Autodesk Fusion 360 part; units mm, degrees
note: some values were not read from the file. Set by a fixed rule: which sketch regions a step uses.
(part 2 of 3)
  arc A535 (3.7573, 18.103) -> (3.7523, 18.103) centre (3.7548, 18.103) ccw
  line L150 (3.7548, 18.103) -> (3.9714, 17.985)
  arc A536 (0.2852, 36.0425) -> (0.2802, 36.0425) centre (0.2827, 36.0425) ccw
  arc A537 (3.5261, 18.189) -> (3.5211, 18.189) centre (3.5236, 18.189) ccw
  arc A538 (3.048, 18.259) -> (3.043, 18.259) centre (3.0455, 18.259) ccw
  line L151 (1.2615, 18.409) -> (1.5123, 18.324)
  line L152 (1.5123, 18.324) -> (1.7721, 18.272)
  arc A539 (0.163, 35.8049) -> (0.168, 35.8049) centre (0.1655, 35.8049) ccw
  arc A540 (2.0389, 18.255) -> (2.0339, 18.255) centre (2.0364, 18.255) ccw
  arc A541 (1.0214, 18.526) -> (1.0264, 18.526) centre (1.0239, 18.526) ccw
  arc A542 (1.7696, 18.272) -> (1.7746, 18.272) centre (1.7721, 18.272) ccw
  arc A543 (0.0779, 35.5541) -> (0.0829, 35.5541) centre (0.0804, 35.5541) ccw
  arc A544 (0.0139, 20.28) -> (0.0089, 20.28) centre (0.0114, 20.28) ccw
  arc A545 (3.5261, 18.189) -> (3.5211, 18.189) centre (3.5236, 18.189) ccw
  arc A546 (3.0389, 18.255) -> (3.0339, 18.255) centre (3.0364, 18.255) ccw
  arc A547 (3.7573, 18.103) -> (3.7523, 18.103) centre (3.7548, 18.103) ccw
  arc A548 (3.043, 18.259) -> (3.048, 18.259) centre (3.0455, 18.259) ccw
  arc A549 (3.0339, 18.255) -> (3.0389, 18.255) centre (3.0364, 18.255) ccw
  arc A550 (1.0264, 18.526) -> (1.0214, 18.526) centre (1.0239, 18.526) ccw
  arc A551 (1.264, 18.409) -> (1.259, 18.409) centre (1.2615, 18.409) ccw
  arc A552 (2.0389, 18.255) -> (2.0339, 18.255) centre (2.0364, 18.255) ccw
  arc A553 (3.9739, 17.985) -> (3.9689, 17.985) centre (3.9714, 17.985) ccw
  arc A554 (3.9689, 17.985) -> (3.9739, 17.985) centre (3.9714, 17.985) ccw
  arc A555 (3.285, 18.242) -> (3.28, 18.242) centre (3.2825, 18.242) ccw
  arc A556 (4.1664, 17.837) -> (4.1714, 17.837) centre (4.1689, 17.837) ccw
  arc A557 (4.1714, 17.837) -> (4.1664, 17.837) centre (4.1689, 17.837) ccw
  arc A558 (0.8012, 18.6735) -> (0.8062, 18.6735) centre (0.8037, 18.6735) ccw
  arc A559 (0.8062, 18.6735) -> (0.8012, 18.6735) centre (0.8037, 18.6735) ccw
  line L153 (3.9714, 17.985) -> (4.1689, 17.837)
  arc A560 (1.259, 18.409) -> (1.264, 18.409) centre (1.2615, 18.409) ccw
  arc A561 (3.9739, 17.985) -> (3.9689, 17.985) centre (3.9714, 17.985) ccw
  arc A562 (4.1714, 17.837) -> (4.1664, 17.837) centre (4.1689, 17.837) ccw
  arc A563 (4.607, 17.248) -> (4.612, 17.248) centre (4.6095, 17.248) ccw
  line L154 (4.6958, 16.043) -> (4.7482, 16.284)
  arc A564 (1.0264, 18.526) -> (1.0214, 18.526) centre (1.0239, 18.526) ccw
  arc A565 (4.3459, 15.397) -> (4.3409, 15.397) centre (4.3434, 15.397) ccw
  arc A566 (4.6933, 17.017) -> (4.6983, 17.017) centre (4.6958, 17.017) ccw
  arc A567 (4.3409, 15.397) -> (4.3459, 15.397) centre (4.3434, 15.397) ccw
  line L155 (3.0455, 18.259) -> (3.2825, 18.242)
  arc A568 (1.5148, 18.324) -> (1.5098, 18.324) centre (1.5123, 18.324) ccw
  arc A569 (1.7696, 18.272) -> (1.7746, 18.272) centre (1.7721, 18.272) ccw
  arc A570 (1.5098, 18.324) -> (1.5148, 18.324) centre (1.5123, 18.324) ccw
  arc A571 (4.6983, 17.017) -> (4.6933, 17.017) centre (4.6958, 17.017) ccw
  arc A572 (4.607, 15.812) -> (4.612, 15.812) centre (4.6095, 15.812) ccw
  arc A573 (4.6983, 16.043) -> (4.6933, 16.043) centre (4.6958, 16.043) ccw
  arc A574 (4.1664, 15.223) -> (4.1714, 15.223) centre (4.1689, 15.223) ccw
  arc A575 (4.7633, 16.53) -> (4.7683, 16.53) centre (4.7658, 16.53) ccw
  arc A576 (3.28, 18.242) -> (3.285, 18.242) centre (3.2825, 18.242) ccw
  line L156 (4.7482, 16.776) -> (4.7658, 16.53)
  arc A577 (4.607, 15.812) -> (4.612, 15.812) centre (4.6095, 15.812) ccw
  arc A578 (0.602, 18.8481) -> (0.607, 18.8481) centre (0.6045, 18.8481) ccw
  arc A579 (4.7683, 16.53) -> (4.7633, 16.53) centre (4.7658, 16.53) ccw
  arc A580 (4.7507, 16.776) -> (4.7457, 16.776) centre (4.7482, 16.776) ccw
  arc A581 (4.4938, 15.595) -> (4.4888, 15.595) centre (4.4913, 15.595) ccw
  arc A582 (4.3409, 17.663) -> (4.3459, 17.663) centre (4.3434, 17.663) ccw
  arc A583 (3.9739, 15.075) -> (3.9689, 15.075) centre (3.9714, 15.075) ccw
  line L157 (4.4913, 15.595) -> (4.6095, 15.812)
  arc A584 (4.1664, 15.223) -> (4.1714, 15.223) centre (4.1689, 15.223) ccw
  arc A585 (4.6933, 16.043) -> (4.6983, 16.043) centre (4.6958, 16.043) ccw
  arc A586 (4.4888, 15.595) -> (4.4938, 15.595) centre (4.4913, 15.595) ccw
  arc A587 (4.7683, 16.53) -> (4.7633, 16.53) centre (4.7658, 16.53) ccw
  arc A588 (4.3409, 15.397) -> (4.3459, 15.397) centre (4.3434, 15.397) ccw
  line L158 (4.4913, 17.465) -> (4.6095, 17.248)
  arc A589 (2.0339, 18.255) -> (2.0389, 18.255) centre (2.0364, 18.255) ccw
  line L159 (3.2825, 18.242) -> (3.5236, 18.189)
  arc A590 (4.7457, 16.776) -> (4.7507, 16.776) centre (4.7482, 16.776) ccw
  arc A591 (4.4888, 15.595) -> (4.4938, 15.595) centre (4.4913, 15.595) ccw
  line L160 (4.6095, 17.248) -> (4.6958, 17.017)
  arc A592 (4.7633, 16.53) -> (4.7683, 16.53) centre (4.7658, 16.53) ccw
  arc A593 (4.612, 17.248) -> (4.607, 17.248) centre (4.6095, 17.248) ccw
  arc A594 (4.7507, 16.284) -> (4.7457, 16.284) centre (4.7482, 16.284) ccw
  arc A595 (4.4938, 17.465) -> (4.4888, 17.465) centre (4.4913, 17.465) ccw
  line L161 (4.3434, 17.663) -> (4.4913, 17.465)
  arc A596 (4.6983, 17.017) -> (4.6933, 17.017) centre (4.6958, 17.017) ccw
  arc A597 (4.6933, 17.017) -> (4.6983, 17.017) centre (4.6958, 17.017) ccw
  line L162 (4.1689, 17.837) -> (4.3434, 17.663)
  arc A598 (4.7507, 16.284) -> (4.7457, 16.284) centre (4.7482, 16.284) ccw
  arc A599 (4.4938, 15.595) -> (4.4888, 15.595) centre (4.4913, 15.595) ccw
  arc A600 (4.3459, 15.397) -> (4.3409, 15.397) centre (4.3434, 15.397) ccw
  arc A601 (4.1714, 15.223) -> (4.1664, 15.223) centre (4.1689, 15.223) ccw
  arc A602 (4.612, 15.812) -> (4.607, 15.812) centre (4.6095, 15.812) ccw
  arc A603 (4.612, 15.812) -> (4.607, 15.812) centre (4.6095, 15.812) ccw
  line L163 (3.9714, 15.075) -> (4.1689, 15.223)
  arc A604 (3.9689, 15.075) -> (3.9739, 15.075) centre (3.9714, 15.075) ccw
  arc A605 (4.4888, 17.465) -> (4.4938, 17.465) centre (4.4913, 17.465) ccw
  arc A606 (3.28, 18.242) -> (3.285, 18.242) centre (3.2825, 18.242) ccw
  line L164 (4.3434, 15.397) -> (4.4913, 15.595)
  arc A607 (4.3409, 17.663) -> (4.3459, 17.663) centre (4.3434, 17.663) ccw
  arc A608 (4.3459, 17.663) -> (4.3409, 17.663) centre (4.3434, 17.663) ccw
  arc A609 (4.7457, 16.284) -> (4.7507, 16.284) centre (4.7482, 16.284) ccw
  arc A610 (4.612, 17.248) -> (4.607, 17.248) centre (4.6095, 17.248) ccw
  arc A611 (4.4888, 17.465) -> (4.4938, 17.465) centre (4.4913, 17.465) ccw
  line L165 (4.6095, 15.812) -> (4.6958, 16.043)
  arc A612 (3.285, 18.242) -> (3.28, 18.242) centre (3.2825, 18.242) ccw
  line L166 (4.1689, 15.223) -> (4.3434, 15.397)
  arc A613 (4.4938, 17.465) -> (4.4888, 17.465) centre (4.4913, 17.465) ccw
  line L167 (4.7482, 16.284) -> (4.7658, 16.53)
  arc A614 (4.3459, 17.663) -> (4.3409, 17.663) centre (4.3434, 17.663) ccw
  arc A615 (4.7457, 16.284) -> (4.7507, 16.284) centre (4.7482, 16.284) ccw
  arc A616 (4.607, 17.248) -> (4.612, 17.248) centre (4.6095, 17.248) ccw
  arc A617 (4.6983, 16.043) -> (4.6933, 16.043) centre (4.6958, 16.043) ccw
  line L168 (4.6958, 17.017) -> (4.7482, 16.776)
  arc A618 (4.7507, 16.776) -> (4.7457, 16.776) centre (4.7482, 16.776) ccw
  arc A619 (4.7457, 16.776) -> (4.7507, 16.776) centre (4.7482, 16.776) ccw
  arc A620 (4.1664, 17.837) -> (4.1714, 17.837) centre (4.1689, 17.837) ccw
  arc A621 (4.6933, 16.043) -> (4.6983, 16.043) centre (4.6958, 16.043) ccw
  line L169 (1.2615, 14.651) -> (1.5123, 14.736)
  arc A622 (1.259, 14.651) -> (1.264, 14.651) centre (1.2615, 14.651) ccw
  arc A623 (1.5098, 14.736) -> (1.5148, 14.736) centre (1.5123, 14.736) ccw
  arc A624 (3.7573, 14.957) -> (3.7523, 14.957) centre (3.7548, 14.957) ccw
  arc A625 (1.7746, 14.788) -> (1.7696, 14.788) centre (1.7721, 14.788) ccw
  arc A626 (2.0389, 14.805) -> (2.0339, 14.805) centre (2.0364, 14.805) ccw
  arc A627 (1.5148, 14.736) -> (1.5098, 14.736) centre (1.5123, 14.736) ccw
  arc A628 (1.259, 14.651) -> (1.264, 14.651) centre (1.2615, 14.651) ccw
  arc A629 (0.8062, 14.387) -> (0.8012, 14.387) centre (0.8037, 14.387) ccw
  arc A630 (56.082, 29.6125) -> (56.077, 29.6125) centre (56.0795, 29.6125) ccw
  arc A631 (56.2584, 29.5441) -> (56.2534, 29.5441) centre (56.2559, 29.5441) ccw
  arc A632 (56.4393, 29.5094) -> (56.4443, 29.5094) centre (56.4418, 29.5094) ccw
  arc A633 (55.5089, 30.53) -> (55.5139, 30.53) centre (55.5114, 30.53) ccw
  arc A634 (56.4393, 29.5094) -> (56.4443, 29.5094) centre (56.4418, 29.5094) ccw
  arc A635 (55.5139, 32.53) -> (55.5089, 32.53) centre (55.5114, 32.53) ccw
  arc A636 (56.4443, 29.5094) -> (56.4393, 29.5094) centre (56.4418, 29.5094) ccw
  line L170 (55.5289, 32.7183) -> (55.5806, 32.9003)
  line L171 (55.5114, 32.53) -> (55.5289, 32.7183)
  arc A637 (55.6624, 33.0696) -> (55.6674, 33.0696) centre (55.6649, 33.0696) ccw
  arc A638 (55.5831, 32.9003) -> (55.5781, 32.9003) centre (55.5806, 32.9003) ccw
  arc A639 (55.5781, 30.1597) -> (55.5831, 30.1597) centre (55.5806, 30.1597) ccw
  arc A640 (55.7814, 29.8395) -> (55.7764, 29.8395) centre (55.7789, 29.8395) ccw
  arc A641 (55.7764, 29.8395) -> (55.7814, 29.8395) centre (55.7789, 29.8395) ccw
  arc A642 (55.5831, 30.1597) -> (55.5781, 30.1597) centre (55.5806, 30.1597) ccw
  arc A643 (55.6674, 29.9904) -> (55.6624, 29.9904) centre (55.6649, 29.9904) ccw
  arc A644 (55.5139, 30.53) -> (55.5089, 30.53) centre (55.5114, 30.53) ccw
  arc A645 (55.5139, 30.53) -> (55.5089, 30.53) centre (55.5114, 30.53) ccw
  arc A646 (55.5314, 32.7183) -> (55.5264, 32.7183) centre (55.5289, 32.7183) ccw
  arc A647 (55.5831, 30.1597) -> (55.5781, 30.1597) centre (55.5806, 30.1597) ccw
  arc A648 (55.6624, 29.9904) -> (55.6674, 29.9904) centre (55.6649, 29.9904) ccw
  arc A649 (55.6674, 29.9904) -> (55.6624, 29.9904) centre (55.6649, 29.9904) ccw
  line L172 (55.6649, 29.9904) -> (55.7789, 29.8395)
  line L173 (55.9187, 29.712) -> (56.0795, 29.6125)
  arc A650 (56.077, 29.6125) -> (56.082, 29.6125) centre (56.0795, 29.6125) ccw
  line L174 (56.4418, 29.5094) -> (56.631, 29.5094)
  arc A651 (55.5314, 30.3417) -> (55.5264, 30.3417) centre (55.5289, 30.3417) ccw
  arc A652 (55.6624, 29.9904) -> (55.6674, 29.9904) centre (55.6649, 29.9904) ccw
  arc A653 (55.5139, 32.53) -> (55.5089, 32.53) centre (55.5114, 32.53) ccw
  line L175 (55.5114, 30.53) -> (55.5114, 32.53)
  arc A654 (55.5089, 32.53) -> (55.5139, 32.53) centre (55.5114, 32.53) ccw
  arc A655 (55.5264, 32.7183) -> (55.5314, 32.7183) centre (55.5289, 32.7183) ccw
  arc A656 (55.7764, 29.8395) -> (55.7814, 29.8395) centre (55.7789, 29.8395) ccw
  arc A657 (55.5264, 30.3417) -> (55.5314, 30.3417) centre (55.5289, 30.3417) ccw
  arc A658 (55.5314, 32.7183) -> (55.5264, 32.7183) centre (55.5289, 32.7183) ccw
  line L176 (55.7789, 29.8395) -> (55.9187, 29.712)
  arc A659 (55.7814, 29.8395) -> (55.7764, 29.8395) centre (55.7789, 29.8395) ccw
  line L177 (55.5289, 30.3417) -> (55.5806, 30.1597)
  arc A660 (56.2534, 29.5441) -> (56.2584, 29.5441) centre (56.2559, 29.5441) ccw
  arc A661 (56.4443, 29.5094) -> (56.4393, 29.5094) centre (56.4418, 29.5094) ccw
  line L178 (55.5806, 30.1597) -> (55.6649, 29.9904)
  line L179 (55.5114, 30.53) -> (55.5289, 30.3417)
  arc A662 (55.5781, 30.1597) -> (55.5831, 30.1597) centre (55.5806, 30.1597) ccw
  arc A663 (55.9162, 29.712) -> (55.9212, 29.712) centre (55.9187, 29.712) ccw
  arc A664 (55.9212, 29.712) -> (55.9162, 29.712) centre (55.9187, 29.712) ccw
  arc A665 (56.6335, 29.5094) -> (56.6285, 29.5094) centre (56.631, 29.5094) ccw
  arc A666 (56.6285, 29.5094) -> (56.6335, 29.5094) centre (56.631, 29.5094) ccw
  line L180 (56.2559, 29.5441) -> (56.4418, 29.5094)
  arc A667 (56.082, 29.6125) -> (56.077, 29.6125) centre (56.0795, 29.6125) ccw
  arc A668 (55.9212, 29.712) -> (55.9162, 29.712) centre (55.9187, 29.712) ccw
  arc A669 (56.2534, 29.5441) -> (56.2584, 29.5441) centre (56.2559, 29.5441) ccw
  arc A670 (55.5314, 30.3417) -> (55.5264, 30.3417) centre (55.5289, 30.3417) ccw
  line L181 (55.5806, 32.9003) -> (55.6649, 33.0696)
  arc A671 (55.5264, 30.3417) -> (55.5314, 30.3417) centre (55.5289, 30.3417) ccw
  arc A672 (55.5089, 30.53) -> (55.5139, 30.53) centre (55.5114, 30.53) ccw
  arc A673 (56.2584, 29.5441) -> (56.2534, 29.5441) centre (56.2559, 29.5441) ccw
  arc A674 (56.6285, 29.5094) -> (56.6335, 29.5094) centre (56.631, 29.5094) ccw
  arc A675 (55.9162, 29.712) -> (55.9212, 29.712) centre (55.9187, 29.712) ccw
  arc A676 (56.077, 29.6125) -> (56.082, 29.6125) centre (56.0795, 29.6125) ccw
  line L182 (56.631, 29.5094) -> (56.8169, 29.5441)
  arc A677 (55.5089, 32.53) -> (55.5139, 32.53) centre (55.5114, 32.53) ccw
  line L183 (56.0795, 29.6125) -> (56.2559, 29.5441)
  arc A678 (57.2914, 29.8395) -> (57.2964, 29.8395) centre (57.2939, 29.8395) ccw
  arc A679 (57.2964, 29.8395) -> (57.2914, 29.8395) centre (57.2939, 29.8395) ccw
  arc A680 (57.4897, 30.1597) -> (57.4947, 30.1597) centre (57.4922, 30.1597) ccw
  arc A681 (57.1566, 29.712) -> (57.1516, 29.712) centre (57.1541, 29.712) ccw
  arc A682 (57.4104, 29.9904) -> (57.4054, 29.9904) centre (57.4079, 29.9904) ccw
  arc A683 (57.4947, 30.1597) -> (57.4897, 30.1597) centre (57.4922, 30.1597) ccw
  arc A684 (57.5464, 30.3417) -> (57.5414, 30.3417) centre (57.5439, 30.3417) ccw
  arc A685 (57.1516, 29.712) -> (57.1566, 29.712) centre (57.1541, 29.712) ccw
  arc A686 (107.0509, 0.276) -> (107.0459, 0.276) centre (107.0484, 0.276) ccw
  arc A687 (64.5089, 30.53) -> (64.5139, 30.53) centre (64.5114, 30.53) ccw
  arc A688 (57.1516, 29.712) -> (57.1566, 29.712) centre (57.1541, 29.712) ccw
  arc A689 (117.4659, 17.248) -> (117.4609, 17.248) centre (117.4634, 17.248) ccw
  line L184 (57.2939, 29.8395) -> (57.4079, 29.9904)
  arc A690 (117.5789, 17.465) -> (117.5839, 17.465) centre (117.5814, 17.465) ccw
  arc A691 (117.5839, 17.465) -> (117.5789, 17.465) centre (117.5814, 17.465) ccw
  arc A692 (56.9958, 29.6125) -> (56.9908, 29.6125) centre (56.9933, 29.6125) ccw
  line L185 (56.631, 33.5506) -> (56.8169, 33.5159)
  arc A693 (56.8144, 29.5441) -> (56.8194, 29.5441) centre (56.8169, 29.5441) ccw
  arc A694 (57.4104, 29.9904) -> (57.4054, 29.9904) centre (57.4079, 29.9904) ccw
  arc A695 (56.6285, 33.5506) -> (56.6335, 33.5506) centre (56.631, 33.5506) ccw
  arc A696 (56.6335, 33.5506) -> (56.6285, 33.5506) centre (56.631, 33.5506) ccw
  arc A697 (56.8144, 33.5159) -> (56.8194, 33.5159) centre (56.8169, 33.5159) ccw
  arc A698 (57.4054, 29.9904) -> (57.4104, 29.9904) centre (57.4079, 29.9904) ccw
  arc A699 (57.4897, 30.1597) -> (57.4947, 30.1597) centre (57.4922, 30.1597) ccw
  arc A700 (57.4947, 30.1597) -> (57.4897, 30.1597) centre (57.4922, 30.1597) ccw
  line L186 (57.5439, 30.3417) -> (57.5614, 30.53)
  arc A701 (57.2964, 29.8395) -> (57.2914, 29.8395) centre (57.2939, 29.8395) ccw
  line L187 (57.4922, 30.1597) -> (57.5439, 30.3417)
  line L188 (107.0484, 0.276) -> (107.2694, 0.423)
  arc A702 (57.5414, 30.3417) -> (57.5464, 30.3417) centre (57.5439, 30.3417) ccw
  line L189 (57.4079, 29.9904) -> (57.4922, 30.1597)
  arc A703 (56.9908, 29.6125) -> (56.9958, 29.6125) centre (56.9933, 29.6125) ccw
  arc A704 (57.1566, 29.712) -> (57.1516, 29.712) centre (57.1541, 29.712) ccw
  arc A705 (57.2914, 29.8395) -> (57.2964, 29.8395) centre (57.2939, 29.8395) ccw
  arc A706 (56.9908, 29.6125) -> (56.9958, 29.6125) centre (56.9933, 29.6125) ccw
  line L190 (56.9933, 29.6125) -> (57.1541, 29.712)
  arc A707 (56.8194, 29.5441) -> (56.8144, 29.5441) centre (56.8169, 29.5441) ccw
  line L191 (64.5114, 30.53) -> (64.5114, 32.53)
  arc A708 (56.8144, 29.5441) -> (56.8194, 29.5441) centre (56.8169, 29.5441) ccw
  line L192 (56.8169, 29.5441) -> (56.9933, 29.6125)
  arc A709 (56.9958, 29.6125) -> (56.9908, 29.6125) centre (56.9933, 29.6125) ccw
  arc A710 (107.2669, 0.423) -> (107.2719, 0.423) centre (107.2694, 0.423) ccw
  arc A711 (64.5139, 30.53) -> (64.5089, 30.53) centre (64.5114, 30.53) ccw
  arc A712 (107.2719, 0.423) -> (107.2669, 0.423) centre (107.2694, 0.423) ccw
  arc A713 (57.4054, 29.9904) -> (57.4104, 29.9904) centre (57.4079, 29.9904) ccw
  arc A714 (107.0459, 0.276) -> (107.0509, 0.276) centre (107.0484, 0.276) ccw
  arc A715 (64.5309, 32.7183) -> (64.5259, 32.7183) centre (64.5284, 32.7183) ccw
  line L193 (117.4634, 17.248) -> (117.5814, 17.465)
  arc A716 (56.6335, 29.5094) -> (56.6285, 29.5094) centre (56.631, 29.5094) ccw
  arc A717 (117.4609, 17.248) -> (117.4659, 17.248) centre (117.4634, 17.248) ccw
  line L194 (57.1541, 29.712) -> (57.2939, 29.8395)
  arc A718 (56.8194, 29.5441) -> (56.8144, 29.5441) centre (56.8169, 29.5441) ccw
  arc A719 (108.0639, 3.03) -> (108.0589, 3.03) centre (108.0614, 3.03) ccw
  arc A720 (108.0589, 2.03) -> (108.0639, 2.03) centre (108.0614, 2.03) ccw
  arc A721 (110.0299, 5.009) -> (110.0249, 5.009) centre (110.0274, 5.009) ccw
  arc A722 (108.0549, 3.039) -> (108.0599, 3.039) centre (108.0574, 3.039) ccw
  arc A723 (108.0599, 3.039) -> (108.0549, 3.039) centre (108.0574, 3.039) ccw
  arc A724 (108.0549, 3.039) -> (108.0599, 3.039) centre (108.0574, 3.039) ccw
  arc A725 (109.0439, 4.744) -> (109.0489, 4.744) centre (109.0464, 4.744) ccw
  arc A726 (113.0339, 5.005) -> (113.0389, 5.005) centre (113.0364, 5.005) ccw
  arc A727 (108.0589, 2.03) -> (108.0639, 2.03) centre (108.0614, 2.03) ccw
  arc A728 (108.4639, 4.235) -> (108.4689, 4.235) centre (108.4664, 4.235) ccw
  line L195 (107.9074, 1.255) -> (107.9924, 1.506)
  arc A729 (108.0589, 3.03) -> (108.0639, 3.03) centre (108.0614, 3.03) ccw
  arc A730 (107.9099, 1.255) -> (107.9049, 1.255) centre (107.9074, 1.255) ccw
  arc A731 (108.4689, 4.235) -> (108.4639, 4.235) centre (108.4664, 4.235) ccw
  arc A732 (108.0639, 2.03) -> (108.0589, 2.03) centre (108.0614, 2.03) ccw
  arc A733 (107.7879, 1.018) -> (107.7929, 1.018) centre (107.7904, 1.018) ccw
  line L196 (108.0614, 2.03) -> (108.0614, 3.03)
  arc A734 (108.0639, 3.03) -> (108.0589, 3.03) centre (108.0614, 3.03) ccw
  arc A735 (113.0479, 5.009) -> (113.0429, 5.009) centre (113.0454, 5.009) ccw
  arc A736 (108.2099, 3.787) -> (108.2049, 3.787) centre (108.2074, 3.787) ccw
  arc A737 (109.0439, 4.744) -> (109.0489, 4.744) centre (109.0464, 4.744) ccw
  arc A738 (109.5219, 4.942) -> (109.5269, 4.942) centre (109.5244, 4.942) ccw
  arc A739 (108.4639, 4.235) -> (108.4689, 4.235) centre (108.4664, 4.235) ccw
  arc A740 (109.0489, 4.744) -> (109.0439, 4.744) centre (109.0464, 4.744) ccw
  line L197 (110.0274, 5.009) -> (110.0364, 5.005)
  arc A741 (108.0639, 2.03) -> (108.0589, 2.03) centre (108.0614, 2.03) ccw
  arc A742 (110.0249, 5.009) -> (110.0299, 5.009) centre (110.0274, 5.009) ccw
  arc A743 (108.3199, 4.02) -> (108.3249, 4.02) centre (108.3224, 4.02) ccw
  arc A744 (108.4689, 4.235) -> (108.4639, 4.235) centre (108.4664, 4.235) ccw
  arc A745 (108.6389, 4.43) -> (108.6339, 4.43) centre (108.6364, 4.43) ccw
  arc A746 (107.9049, 1.255) -> (107.9099, 1.255) centre (107.9074, 1.255) ccw
  arc A747 (107.9949, 1.506) -> (107.9899, 1.506) centre (107.9924, 1.506) ccw
  line L198 (108.0744, 3.288) -> (108.1244, 3.542)
  arc A748 (108.1219, 3.542) -> (108.1269, 3.542) centre (108.1244, 3.542) ccw
  arc A749 (110.0339, 5.005) -> (110.0389, 5.005) centre (110.0364, 5.005) ccw
  line L199 (109.7784, 4.992) -> (110.0274, 5.009)
  arc A750 (107.9899, 1.506) -> (107.9949, 1.506) centre (107.9924, 1.506) ccw
  line L200 (113.2944, 4.992) -> (113.5484, 4.942)
  arc A751 (108.0419, 1.766) -> (108.0469, 1.766) centre (108.0444, 1.766) ccw
  arc A752 (107.9099, 1.255) -> (107.9049, 1.255) centre (107.9074, 1.255) ccw
  arc A753 (108.0589, 3.03) -> (108.0639, 3.03) centre (108.0614, 3.03) ccw
  line L201 (107.9924, 1.506) -> (108.0444, 1.766)
  arc A754 (108.1269, 3.542) -> (108.1219, 3.542) centre (108.1244, 3.542) ccw
  arc A755 (107.9899, 1.506) -> (107.9949, 1.506) centre (107.9924, 1.506) ccw
  line L202 (108.2074, 3.787) -> (108.3224, 4.02)
  arc A756 (108.2049, 3.787) -> (108.2099, 3.787) centre (108.2074, 3.787) ccw
  line L203 (108.3224, 4.02) -> (108.4664, 4.235)
  line L204 (108.1244, 3.542) -> (108.2074, 3.787)
  arc A757 (108.3249, 4.02) -> (108.3199, 4.02) centre (108.3224, 4.02) ccw
  arc A758 (108.3249, 4.02) -> (108.3199, 4.02) centre (108.3224, 4.02) ccw
  arc A759 (107.7929, 1.018) -> (107.7879, 1.018) centre (107.7904, 1.018) ccw
  line L205 (108.4664, 4.235) -> (108.6364, 4.43)
  arc A760 (107.7929, 1.018) -> (107.7879, 1.018) centre (107.7904, 1.018) ccw
  arc A761 (108.0419, 1.766) -> (108.0469, 1.766) centre (108.0444, 1.766) ccw
  arc A762 (113.2919, 4.992) -> (113.2969, 4.992) centre (113.2944, 4.992) ccw
  arc A763 (108.6339, 4.43) -> (108.6389, 4.43) centre (108.6364, 4.43) ccw
  arc A764 (108.0769, 3.288) -> (108.0719, 3.288) centre (108.0744, 3.288) ccw
  arc A765 (107.9049, 1.255) -> (107.9099, 1.255) centre (107.9074, 1.255) ccw
  arc A766 (108.3199, 4.02) -> (108.3249, 4.02) centre (108.3224, 4.02) ccw
  arc A767 (108.8289, 4.6) -> (108.8339, 4.6) centre (108.8314, 4.6) ccw
  arc A768 (110.0389, 5.005) -> (110.0339, 5.005) centre (110.0364, 5.005) ccw
  arc A769 (109.0489, 4.744) -> (109.0439, 4.744) centre (109.0464, 4.744) ccw
  arc A770 (114.0239, 4.744) -> (114.0289, 4.744) centre (114.0264, 4.744) ccw
  arc A771 (109.2769, 4.859) -> (109.2819, 4.859) centre (109.2794, 4.859) ccw
  arc A772 (113.7909, 4.859) -> (113.7959, 4.859) centre (113.7934, 4.859) ccw
  arc A773 (109.2819, 4.859) -> (109.2769, 4.859) centre (109.2794, 4.859) ccw
  line L206 (113.0454, 5.009) -> (113.2944, 4.992)
  arc A774 (109.7809, 4.992) -> (109.7759, 4.992) centre (109.7784, 4.992) ccw
  line L207 (109.2794, 4.859) -> (109.5244, 4.942)
  arc A775 (109.5269, 4.942) -> (109.5219, 4.942) centre (109.5244, 4.942) ccw
  arc A776 (109.7809, 4.992) -> (109.7759, 4.992) centre (109.7784, 4.992) ccw
  arc A777 (109.5269, 4.942) -> (109.5219, 4.942) centre (109.5244, 4.942) ccw
  arc A778 (110.0389, 5.005) -> (110.0339, 5.005) centre (110.0364, 5.005) ccw
  arc A779 (110.0299, 5.009) -> (110.0249, 5.009) centre (110.0274, 5.009) ccw
  arc A780 (108.6389, 4.43) -> (108.6339, 4.43) centre (108.6364, 4.43) ccw
  arc A781 (113.5459, 4.942) -> (113.5509, 4.942) centre (113.5484, 4.942) ccw
  arc A782 (113.7959, 4.859) -> (113.7909, 4.859) centre (113.7934, 4.859) ccw
  arc A783 (113.0429, 5.009) -> (113.0479, 5.009) centre (113.0454, 5.009) ccw
  arc A784 (114.2439, 4.6) -> (114.2389, 4.6) centre (114.2414, 4.6) ccw
  arc A785 (113.2969, 4.992) -> (113.2919, 4.992) centre (113.2944, 4.992) ccw
  arc A786 (114.4339, 4.43) -> (114.4389, 4.43) centre (114.4364, 4.43) ccw
  arc A787 (114.7479, 4.02) -> (114.7529, 4.02) centre (114.7504, 4.02) ccw
  arc A788 (115.0009, 3.288) -> (114.9959, 3.288) centre (114.9984, 3.288) ccw
  arc A789 (114.9959, 3.288) -> (115.0009, 3.288) centre (114.9984, 3.288) ccw
  arc A790 (113.0429, 5.009) -> (113.0479, 5.009) centre (113.0454, 5.009) ccw
  arc A791 (108.8339, 4.6) -> (108.8289, 4.6) centre (108.8314, 4.6) ccw
  arc A792 (113.0389, 5.005) -> (113.0339, 5.005) centre (113.0364, 5.005) ccw
  line L208 (113.5484, 4.942) -> (113.7934, 4.859)
  arc A793 (113.2919, 4.992) -> (113.2969, 4.992) centre (113.2944, 4.992) ccw
  arc A794 (109.5219, 4.942) -> (109.5269, 4.942) centre (109.5244, 4.942) ccw
  arc A795 (113.0479, 5.009) -> (113.0429, 5.009) centre (113.0454, 5.009) ccw
  arc A796 (109.7759, 4.992) -> (109.7809, 4.992) centre (109.7784, 4.992) ccw
  arc A797 (113.5509, 4.942) -> (113.5459, 4.942) centre (113.5484, 4.942) ccw
  line L209 (110.0364, 5.005) -> (113.0364, 5.005)
  arc A798 (109.2819, 4.859) -> (109.2769, 4.859) centre (109.2794, 4.859) ccw
  arc A799 (108.8339, 4.6) -> (108.8289, 4.6) centre (108.8314, 4.6) ccw
  arc A800 (113.7909, 4.859) -> (113.7959, 4.859) centre (113.7934, 4.859) ccw
  arc A801 (108.6339, 4.43) -> (108.6389, 4.43) centre (108.6364, 4.43) ccw
  arc A802 (109.7759, 4.992) -> (109.7809, 4.992) centre (109.7784, 4.992) ccw
  arc A803 (108.8289, 4.6) -> (108.8339, 4.6) centre (108.8314, 4.6) ccw
  arc A804 (110.0339, 5.005) -> (110.0389, 5.005) centre (110.0364, 5.005) ccw
  arc A805 (113.5509, 4.942) -> (113.5459, 4.942) centre (113.5484, 4.942) ccw
  line L210 (109.5244, 4.942) -> (109.7784, 4.992)
  arc A806 (113.2969, 4.992) -> (113.2919, 4.992) centre (113.2944, 4.992) ccw
  arc A807 (113.0389, 5.005) -> (113.0339, 5.005) centre (113.0364, 5.005) ccw
  line L211 (114.6064, 4.235) -> (114.7504, 4.02)
  line L212 (109.0464, 4.744) -> (109.2794, 4.859)
  arc A808 (109.2769, 4.859) -> (109.2819, 4.859) centre (109.2794, 4.859) ccw
  arc A809 (113.0339, 5.005) -> (113.0389, 5.005) centre (113.0364, 5.005) ccw
  arc A810 (114.2389, 4.6) -> (114.2439, 4.6) centre (114.2414, 4.6) ccw
  line L213 (108.6364, 4.43) -> (108.8314, 4.6)
  arc A811 (114.9459, 3.542) -> (114.9509, 3.542) centre (114.9484, 3.542) ccw
  line L214 (113.7934, 4.859) -> (114.0264, 4.744)
  arc A812 (113.5459, 4.942) -> (113.5509, 4.942) centre (113.5484, 4.942) ccw
  arc A813 (113.7959, 4.859) -> (113.7909, 4.859) centre (113.7934, 4.859) ccw
  line L215 (108.8314, 4.6) -> (109.0464, 4.744)
  line L216 (113.0364, 5.005) -> (113.0454, 5.009)
  arc A814 (110.0249, 5.009) -> (110.0299, 5.009) centre (110.0274, 5.009) ccw
  line L217 (114.9984, 3.288) -> (115.0154, 3.039)
  arc A815 (114.9959, 3.288) -> (115.0009, 3.288) centre (114.9984, 3.288) ccw
  arc A816 (115.0089, 3.03) -> (115.0139, 3.03) centre (115.0114, 3.03) ccw
  line L218 (115.0114, 3.03) -> (115.0154, 3.039)
  line L219 (114.2414, 4.6) -> (114.4364, 4.43)
  arc A817 (115.0089, 2.03) -> (115.0139, 2.03) centre (115.0114, 2.03) ccw
  arc A818 (115.0179, 3.039) -> (115.0129, 3.039) centre (115.0154, 3.039) ccw
  arc A819 (114.2439, 4.6) -> (114.2389, 4.6) centre (114.2414, 4.6) ccw
  arc A820 (115.0089, 3.03) -> (115.0139, 3.03) centre (115.0114, 3.03) ccw
  arc A821 (115.0309, 1.766) -> (115.0259, 1.766) centre (115.0284, 1.766) ccw
  arc A822 (114.0289, 4.744) -> (114.0239, 4.744) centre (114.0264, 4.744) ccw
  line L220 (115.0284, 1.766) -> (115.0804, 1.506)
  arc A823 (115.0089, 2.03) -> (115.0139, 2.03) centre (115.0114, 2.03) ccw
  line L221 (115.0804, 1.506) -> (115.1654, 1.255)
  arc A824 (114.6089, 4.235) -> (114.6039, 4.235) centre (114.6064, 4.235) ccw
  arc A825 (114.9509, 3.542) -> (114.9459, 3.542) centre (114.9484, 3.542) ccw
  arc A826 (115.0779, 1.506) -> (115.0829, 1.506) centre (115.0804, 1.506) ccw
  arc A827 (114.0239, 4.744) -> (114.0289, 4.744) centre (114.0264, 4.744) ccw
  arc A828 (114.8679, 3.787) -> (114.8629, 3.787) centre (114.8654, 3.787) ccw
  line L222 (114.4364, 4.43) -> (114.6064, 4.235)
  arc A829 (114.7479, 4.02) -> (114.7529, 4.02) centre (114.7504, 4.02) ccw
  arc A830 (115.0829, 1.506) -> (115.0779, 1.506) centre (115.0804, 1.506) ccw
  line L223 (114.9484, 3.542) -> (114.9984, 3.288)
  arc A831 (115.0179, 3.039) -> (115.0129, 3.039) centre (115.0154, 3.039) ccw
  arc A832 (115.0129, 3.039) -> (115.0179, 3.039) centre (115.0154, 3.039) ccw
  arc A833 (114.4339, 4.43) -> (114.4389, 4.43) centre (114.4364, 4.43) ccw
  arc A834 (114.6039, 4.235) -> (114.6089, 4.235) centre (114.6064, 4.235) ccw
  arc A835 (114.0289, 4.744) -> (114.0239, 4.744) centre (114.0264, 4.744) ccw
  arc A836 (114.8679, 3.787) -> (114.8629, 3.787) centre (114.8654, 3.787) ccw
  line L224 (115.0114, 2.03) -> (115.0114, 3.03)
  arc A837 (115.0139, 3.03) -> (115.0089, 3.03) centre (115.0114, 3.03) ccw
  line L225 (115.0114, 2.03) -> (115.0284, 1.766)
  arc A838 (115.0129, 3.039) -> (115.0179, 3.039) centre (115.0154, 3.039) ccw
  arc A839 (116.5149, 0.074) -> (116.5099, 0.074) centre (116.5124, 0.074) ccw
  arc A840 (116.2589, 0.159) -> (116.2639, 0.159) centre (116.2614, 0.159) ccw
  arc A841 (115.0259, 1.766) -> (115.0309, 1.766) centre (115.0284, 1.766) ccw
  arc A842 (114.4389, 4.43) -> (114.4339, 4.43) centre (114.4364, 4.43) ccw
  arc A843 (115.0779, 1.506) -> (115.0829, 1.506) centre (115.0804, 1.506) ccw
  arc A844 (116.7699, 0.022) -> (116.7749, 0.022) centre (116.7724, 0.022) ccw
  arc A845 (115.0259, 1.766) -> (115.0309, 1.766) centre (115.0284, 1.766) ccw
  arc A846 (114.7529, 4.02) -> (114.7479, 4.02) centre (114.7504, 4.02) ccw
  arc A847 (120.0389, 0.005) -> (120.0339, 0.005) centre (120.0364, 0.005) ccw
  arc A848 (115.2799, 1.018) -> (115.2849, 1.018) centre (115.2824, 1.018) ccw
  arc A849 (120.0339, 0.005) -> (120.0389, 0.005) centre (120.0364, 0.005) ccw
  arc A850 (115.4269, 0.797) -> (115.4319, 0.797) centre (115.4294, 0.797) ccw
  line L226 (114.8654, 3.787) -> (114.9484, 3.542)
  arc A851 (115.0139, 2.03) -> (115.0089, 2.03) centre (115.0114, 2.03) ccw
  arc A852 (114.9459, 3.542) -> (114.9509, 3.542) centre (114.9484, 3.542) ccw
  arc A853 (114.4389, 4.43) -> (114.4339, 4.43) centre (114.4364, 4.43) ccw
  line L227 (114.0264, 4.744) -> (114.2414, 4.6)
  line L228 (114.7504, 4.02) -> (114.8654, 3.787)
  arc A854 (114.9509, 3.542) -> (114.9459, 3.542) centre (114.9484, 3.542) ccw
  arc A855 (114.6089, 4.235) -> (114.6039, 4.235) centre (114.6064, 4.235) ccw
  arc A856 (115.0139, 2.03) -> (115.0089, 2.03) centre (115.0114, 2.03) ccw
  arc A857 (114.6039, 4.235) -> (114.6089, 4.235) centre (114.6064, 4.235) ccw
  arc A858 (115.0009, 3.288) -> (114.9959, 3.288) centre (114.9984, 3.288) ccw
  arc A859 (115.0139, 3.03) -> (115.0089, 3.03) centre (115.0114, 3.03) ccw
  arc A860 (114.2389, 4.6) -> (114.2439, 4.6) centre (114.2414, 4.6) ccw
  arc A861 (115.0309, 1.766) -> (115.0259, 1.766) centre (115.0284, 1.766) ccw
  arc A862 (114.8629, 3.787) -> (114.8679, 3.787) centre (114.8654, 3.787) ccw
  arc A863 (115.0829, 1.506) -> (115.0779, 1.506) centre (115.0804, 1.506) ccw
  arc A864 (114.7529, 4.02) -> (114.7479, 4.02) centre (114.7504, 4.02) ccw
  arc A865 (114.8629, 3.787) -> (114.8679, 3.787) centre (114.8654, 3.787) ccw
  arc A866 (116.0259, 0.276) -> (116.0209, 0.276) centre (116.0234, 0.276) ccw
  arc A867 (117.0389, 0.005) -> (117.0339, 0.005) centre (117.0364, 0.005) ccw
  arc A868 (115.6069, 0.598) -> (115.6019, 0.598) centre (115.6044, 0.598) ccw
  arc A869 (115.2799, 1.018) -> (115.2849, 1.018) centre (115.2824, 1.018) ccw
  arc A870 (120.2979, 0.022) -> (120.3029, 0.022) centre (120.3004, 0.022) ccw
  arc A871 (116.0209, 0.276) -> (116.0259, 0.276) centre (116.0234, 0.276) ccw
  arc A872 (120.5579, 0.074) -> (120.5629, 0.074) centre (120.5604, 0.074) ccw
  line L229 (115.2824, 1.018) -> (115.4294, 0.797)
  line L230 (116.5124, 0.074) -> (116.7724, 0.022)
  arc A873 (116.5099, 0.074) -> (116.5149, 0.074) centre (116.5124, 0.074) ccw
  arc A874 (115.6069, 0.598) -> (115.6019, 0.598) centre (115.6044, 0.598) ccw
  arc A875 (115.8009, 0.423) -> (115.8059, 0.423) centre (115.8034, 0.423) ccw
  line L231 (116.0234, 0.276) -> (116.2614, 0.159)
  line L232 (115.1654, 1.255) -> (115.2824, 1.018)
  arc A876 (117.0389, 0.005) -> (117.0339, 0.005) centre (117.0364, 0.005) ccw
  arc A877 (115.6019, 0.598) -> (115.6069, 0.598) centre (115.6044, 0.598) ccw
  arc A878 (115.4269, 0.797) -> (115.4319, 0.797) centre (115.4294, 0.797) ccw
  arc A879 (115.2849, 1.018) -> (115.2799, 1.018) centre (115.2824, 1.018) ccw
  line L233 (120.0364, 0.005) -> (120.3004, 0.022)
  arc A880 (115.1629, 1.255) -> (115.1679, 1.255) centre (115.1654, 1.255) ccw
  arc A881 (115.1679, 1.255) -> (115.1629, 1.255) centre (115.1654, 1.255) ccw
  arc A882 (116.5099, 0.074) -> (116.5149, 0.074) centre (116.5124, 0.074) ccw
  arc A883 (115.8009, 0.423) -> (115.8059, 0.423) centre (115.8034, 0.423) ccw
  arc A884 (116.7749, 0.022) -> (116.7699, 0.022) centre (116.7724, 0.022) ccw
  line L234 (116.7724, 0.022) -> (117.0364, 0.005)
  line L235 (122.0614, 2.03) -> (122.0614, 12.78)
  arc A885 (120.5629, 0.074) -> (120.5579, 0.074) centre (120.5604, 0.074) ccw
  arc A886 (120.2979, 0.022) -> (120.3029, 0.022) centre (120.3004, 0.022) ccw
  arc A887 (120.3029, 0.022) -> (120.2979, 0.022) centre (120.3004, 0.022) ccw
  line L236 (120.8114, 0.159) -> (121.0484, 0.276)
  line L237 (115.8034, 0.423) -> (116.0234, 0.276)
  arc A888 (115.8059, 0.423) -> (115.8009, 0.423) centre (115.8034, 0.423) ccw
  arc A889 (120.8089, 0.159) -> (120.8139, 0.159) centre (120.8114, 0.159) ccw
  line L238 (120.5604, 0.074) -> (120.8114, 0.159)
  arc A890 (115.4319, 0.797) -> (115.4269, 0.797) centre (115.4294, 0.797) ccw
  arc A891 (120.0339, 0.005) -> (120.0389, 0.005) centre (120.0364, 0.005) ccw
  arc A892 (116.0259, 0.276) -> (116.0209, 0.276) centre (116.0234, 0.276) ccw
  arc A893 (121.4709, 0.598) -> (121.4659, 0.598) centre (121.4684, 0.598) ccw
  arc A894 (120.3029, 0.022) -> (120.2979, 0.022) centre (120.3004, 0.022) ccw
  line L239 (120.3004, 0.022) -> (120.5604, 0.074)
  arc A895 (115.1679, 1.255) -> (115.1629, 1.255) centre (115.1654, 1.255) ccw
  arc A896 (115.1629, 1.255) -> (115.1679, 1.255) centre (115.1654, 1.255) ccw
  arc A897 (120.5629, 0.074) -> (120.5579, 0.074) centre (120.5604, 0.074) ccw
  arc A898 (117.0339, 0.005) -> (117.0389, 0.005) centre (117.0364, 0.005) ccw
  arc A899 (116.2589, 0.159) -> (116.2639, 0.159) centre (116.2614, 0.159) ccw
  arc A900 (116.7699, 0.022) -> (116.7749, 0.022) centre (116.7724, 0.022) ccw
  line L240 (115.6044, 0.598) -> (115.8034, 0.423)
  line L241 (115.4294, 0.797) -> (115.6044, 0.598)
  arc A901 (116.0209, 0.276) -> (116.0259, 0.276) centre (116.0234, 0.276) ccw
  arc A902 (116.7749, 0.022) -> (116.7699, 0.022) centre (116.7724, 0.022) ccw
  arc A903 (116.2639, 0.159) -> (116.2589, 0.159) centre (116.2614, 0.159) ccw
  arc A904 (115.2849, 1.018) -> (115.2799, 1.018) centre (115.2824, 1.018) ccw
  line L242 (117.0364, 0.005) -> (120.0364, 0.005)
  arc A905 (116.2639, 0.159) -> (116.2589, 0.159) centre (116.2614, 0.159) ccw
  arc A906 (122.0469, 1.766) -> (122.0419, 1.766) centre (122.0444, 1.766) ccw
  arc A907 (117.0339, 0.005) -> (117.0389, 0.005) centre (117.0364, 0.005) ccw
  arc A908 (115.8059, 0.423) -> (115.8009, 0.423) centre (115.8034, 0.423) ccw
  arc A909 (120.0389, 0.005) -> (120.0339, 0.005) centre (120.0364, 0.005) ccw
  arc A910 (120.5579, 0.074) -> (120.5629, 0.074) centre (120.5604, 0.074) ccw
  line L243 (116.2614, 0.159) -> (116.5124, 0.074)
  arc A911 (115.4319, 0.797) -> (115.4269, 0.797) centre (115.4294, 0.797) ccw
  arc A912 (115.6019, 0.598) -> (115.6069, 0.598) centre (115.6044, 0.598) ccw
  arc A913 (116.5149, 0.074) -> (116.5099, 0.074) centre (116.5124, 0.074) ccw
  arc A914 (120.8139, 0.159) -> (120.8089, 0.159) centre (120.8114, 0.159) ccw
  arc A915 (121.9049, 1.255) -> (121.9099, 1.255) centre (121.9074, 1.255) ccw
  arc A916 (121.0459, 0.276) -> (121.0509, 0.276) centre (121.0484, 0.276) ccw
  arc A917 (121.6459, 0.797) -> (121.6409, 0.797) centre (121.6434, 0.797) ccw
  arc A918 (121.6409, 0.797) -> (121.6459, 0.797) centre (121.6434, 0.797) ccw
  line L244 (121.9074, 1.255) -> (121.9924, 1.506)
  arc A919 (121.7879, 1.018) -> (121.7929, 1.018) centre (121.7904, 1.018) ccw
  arc A920 (121.0459, 0.276) -> (121.0509, 0.276) centre (121.0484, 0.276) ccw
  arc A921 (122.0469, 13.044) -> (122.0419, 13.044) centre (122.0444, 13.044) ccw
  arc A922 (122.0639, 12.78) -> (122.0589, 12.78) centre (122.0614, 12.78) ccw
  arc A923 (121.6459, 0.797) -> (121.6409, 0.797) centre (121.6434, 0.797) ccw
  arc A924 (121.4659, 0.598) -> (121.4709, 0.598) centre (121.4684, 0.598) ccw
  arc A925 (122.0419, 1.766) -> (122.0469, 1.766) centre (122.0444, 1.766) ccw
  line L245 (121.9924, 13.304) -> (122.0444, 13.044)
  arc A926 (121.9899, 13.304) -> (121.9949, 13.304) centre (121.9924, 13.304) ccw
  arc A927 (122.0639, 2.03) -> (122.0589, 2.03) centre (122.0614, 2.03) ccw
  line L246 (121.7904, 1.018) -> (121.9074, 1.255)
  arc A928 (122.0419, 1.766) -> (122.0469, 1.766) centre (122.0444, 1.766) ccw
  arc A929 (121.9949, 13.304) -> (121.9899, 13.304) centre (121.9924, 13.304) ccw
  arc A930 (122.0639, 12.78) -> (122.0589, 12.78) centre (122.0614, 12.78) ccw
  arc A931 (122.0419, 13.044) -> (122.0469, 13.044) centre (122.0444, 13.044) ccw
  arc A932 (122.0639, 2.03) -> (122.0589, 2.03) centre (122.0614, 2.03) ccw
  arc A933 (121.0509, 0.276) -> (121.0459, 0.276) centre (121.0484, 0.276) ccw
  arc A934 (122.0469, 13.044) -> (122.0419, 13.044) centre (122.0444, 13.044) ccw
  line L247 (121.9074, 13.555) -> (121.9924, 13.304)
  arc A935 (121.9099, 1.255) -> (121.9049, 1.255) centre (121.9074, 1.255) ccw
  arc A936 (122.0589, 2.03) -> (122.0639, 2.03) centre (122.0614, 2.03) ccw
  line L248 (121.2694, 0.423) -> (121.4684, 0.598)
  arc A937 (121.6409, 0.797) -> (121.6459, 0.797) centre (121.6434, 0.797) ccw
  arc A938 (121.7879, 1.018) -> (121.7929, 1.018) centre (121.7904, 1.018) ccw
  arc A939 (121.9899, 1.506) -> (121.9949, 1.506) centre (121.9924, 1.506) ccw
  arc A940 (121.9949, 1.506) -> (121.9899, 1.506) centre (121.9924, 1.506) ccw
  arc A941 (121.2669, 0.423) -> (121.2719, 0.423) centre (121.2694, 0.423) ccw
  arc A942 (120.8139, 0.159) -> (120.8089, 0.159) centre (120.8114, 0.159) ccw
  arc A943 (121.2719, 0.423) -> (121.2669, 0.423) centre (121.2694, 0.423) ccw
  line L249 (121.0484, 0.276) -> (121.2694, 0.423)
  line L250 (122.0444, 1.766) -> (122.0614, 2.03)
  arc A944 (121.2669, 0.423) -> (121.2719, 0.423) centre (121.2694, 0.423) ccw
  arc A945 (121.9099, 1.255) -> (121.9049, 1.255) centre (121.9074, 1.255) ccw
  line L251 (122.0444, 13.044) -> (122.0614, 12.78)
  arc A946 (121.0509, 0.276) -> (121.0459, 0.276) centre (121.0484, 0.276) ccw
  arc A947 (121.9049, 1.255) -> (121.9099, 1.255) centre (121.9074, 1.255) ccw
  arc A948 (122.0469, 1.766) -> (122.0419, 1.766) centre (122.0444, 1.766) ccw
  arc A949 (122.0589, 2.03) -> (122.0639, 2.03) centre (122.0614, 2.03) ccw
  arc A950 (120.2979, 14.788) -> (120.3029, 14.788) centre (120.3004, 14.788) ccw
  arc A951 (121.0509, 14.534) -> (121.0459, 14.534) centre (121.0484, 14.534) ccw
  arc A952 (120.2979, 14.788) -> (120.3029, 14.788) centre (120.3004, 14.788) ccw
  arc A953 (122.0589, 12.78) -> (122.0639, 12.78) centre (122.0614, 12.78) ccw
  line L252 (121.0484, 14.534) -> (121.2694, 14.387)
  arc A954 (121.4709, 0.598) -> (121.4659, 0.598) centre (121.4684, 0.598) ccw
  arc A955 (120.0339, 14.805) -> (120.0389, 14.805) centre (120.0364, 14.805) ccw
  arc A956 (121.6409, 14.013) -> (121.6459, 14.013) centre (121.6434, 14.013) ccw
  arc A957 (121.2719, 14.387) -> (121.2669, 14.387) centre (121.2694, 14.387) ccw
  line L253 (121.9924, 1.506) -> (122.0444, 1.766)
  arc A958 (120.8089, 0.159) -> (120.8139, 0.159) centre (120.8114, 0.159) ccw
  arc A959 (122.0589, 12.78) -> (122.0639, 12.78) centre (122.0614, 12.78) ccw
  arc A960 (121.9899, 1.506) -> (121.9949, 1.506) centre (121.9924, 1.506) ccw
  line L254 (121.4684, 0.598) -> (121.6434, 0.797)
  line L255 (119.0364, 14.805) -> (120.0364, 14.805)
  arc A961 (121.2719, 0.423) -> (121.2669, 0.423) centre (121.2694, 0.423) ccw
  arc A962 (122.0419, 13.044) -> (122.0469, 13.044) centre (122.0444, 13.044) ccw
  arc A963 (121.7929, 1.018) -> (121.7879, 1.018) centre (121.7904, 1.018) ccw
  line L256 (121.6434, 0.797) -> (121.7904, 1.018)
  arc A964 (121.4659, 0.598) -> (121.4709, 0.598) centre (121.4684, 0.598) ccw
  arc A965 (121.9949, 1.506) -> (121.9899, 1.506) centre (121.9924, 1.506) ccw
  arc A966 (121.7929, 1.018) -> (121.7879, 1.018) centre (121.7904, 1.018) ccw
  line L257 (119.0274, 14.801) -> (119.0364, 14.805)
  arc A967 (121.0459, 14.534) -> (121.0509, 14.534) centre (121.0484, 14.534) ccw
  arc A968 (118.5469, 14.871) -> (118.5519, 14.871) centre (118.5494, 14.871) ccw
  arc A969 (120.3029, 14.788) -> (120.2979, 14.788) centre (120.3004, 14.788) ccw
  arc A970 (120.5579, 14.736) -> (120.5629, 14.736) centre (120.5604, 14.736) ccw
  arc A971 (120.8139, 14.651) -> (120.8089, 14.651) centre (120.8114, 14.651) ccw
  arc A972 (117.3749, 16.043) -> (117.3799, 16.043) centre (117.3774, 16.043) ccw
  arc A973 (121.9099, 13.555) -> (121.9049, 13.555) centre (121.9074, 13.555) ccw
  arc A974 (119.0389, 14.805) -> (119.0339, 14.805) centre (119.0364, 14.805) ccw
  arc A975 (118.7879, 14.818) -> (118.7929, 14.818) centre (118.7904, 14.818) ccw
  arc A976 (120.5629, 14.736) -> (120.5579, 14.736) centre (120.5604, 14.736) ccw
  arc A977 (121.6459, 14.013) -> (121.6409, 14.013) centre (121.6434, 14.013) ccw
  line L258 (118.7904, 14.818) -> (119.0274, 14.801)
  arc A978 (121.9049, 13.555) -> (121.9099, 13.555) centre (121.9074, 13.555) ccw
  line L259 (121.7904, 13.793) -> (121.9074, 13.555)
  arc A979 (121.4709, 14.212) -> (121.4659, 14.212) centre (121.4684, 14.212) ccw
  arc A980 (121.6409, 14.013) -> (121.6459, 14.013) centre (121.6434, 14.013) ccw
  arc A981 (119.0339, 14.805) -> (119.0389, 14.805) centre (119.0364, 14.805) ccw
  line L260 (120.8114, 14.651) -> (121.0484, 14.534)
  arc A982 (119.0299, 14.801) -> (119.0249, 14.801) centre (119.0274, 14.801) ccw
  arc A983 (119.0249, 14.801) -> (119.0299, 14.801) centre (119.0274, 14.801) ccw
  arc A984 (119.0249, 14.801) -> (119.0299, 14.801) centre (119.0274, 14.801) ccw
  arc A985 (120.5579, 14.736) -> (120.5629, 14.736) centre (120.5604, 14.736) ccw
  line L261 (120.3004, 14.788) -> (120.5604, 14.736)
  arc A986 (121.4709, 14.212) -> (121.4659, 14.212) centre (121.4684, 14.212) ccw
  arc A987 (120.8089, 14.651) -> (120.8139, 14.651) centre (120.8114, 14.651) ccw
  arc A988 (121.7879, 13.793) -> (121.7929, 13.793) centre (121.7904, 13.793) ccw
  arc A989 (121.9949, 13.304) -> (121.9899, 13.304) centre (121.9924, 13.304) ccw
  arc A990 (121.2669, 14.387) -> (121.2719, 14.387) centre (121.2694, 14.387) ccw
  line L262 (120.5604, 14.736) -> (120.8114, 14.651)
  arc A991 (121.7929, 13.793) -> (121.7879, 13.793) centre (121.7904, 13.793) ccw
  arc A992 (120.8139, 14.651) -> (120.8089, 14.651) centre (120.8114, 14.651) ccw
  arc A993 (121.6459, 14.013) -> (121.6409, 14.013) centre (121.6434, 14.013) ccw
  line L263 (120.0364, 14.805) -> (120.3004, 14.788)
  arc A994 (120.5629, 14.736) -> (120.5579, 14.736) centre (120.5604, 14.736) ccw
  arc A995 (118.7929, 14.818) -> (118.7879, 14.818) centre (118.7904, 14.818) ccw
  arc A996 (120.3029, 14.788) -> (120.2979, 14.788) centre (120.3004, 14.788) ccw
  line L264 (121.4684, 14.212) -> (121.6434, 14.013)
  arc A997 (118.7879, 14.818) -> (118.7929, 14.818) centre (118.7904, 14.818) ccw
  arc A998 (121.2669, 14.387) -> (121.2719, 14.387) centre (121.2694, 14.387) ccw
  arc A999 (120.0389, 14.805) -> (120.0339, 14.805) centre (120.0364, 14.805) ccw
  line L265 (121.2694, 14.387) -> (121.4684, 14.212)
  arc A1000 (121.9899, 13.304) -> (121.9949, 13.304) centre (121.9924, 13.304) ccw
  arc A1001 (121.7879, 13.793) -> (121.7929, 13.793) centre (121.7904, 13.793) ccw
  line L266 (121.6434, 14.013) -> (121.7904, 13.793)
  arc A1002 (119.0389, 14.805) -> (119.0339, 14.805) centre (119.0364, 14.805) ccw
  arc A1003 (119.0339, 14.805) -> (119.0389, 14.805) centre (119.0364, 14.805) ccw
  arc A1004 (120.0389, 14.805) -> (120.0339, 14.805) centre (120.0364, 14.805) ccw
  arc A1005 (117.4609, 15.812) -> (117.4659, 15.812) centre (117.4634, 15.812) ccw
  arc A1006 (121.0459, 14.534) -> (121.0509, 14.534) centre (121.0484, 14.534) ccw
  arc A1007 (121.9049, 13.555) -> (121.9099, 13.555) centre (121.9074, 13.555) ccw
  arc A1008 (120.0339, 14.805) -> (120.0389, 14.805) centre (120.0364, 14.805) ccw
  arc A1009 (118.3209, 14.957) -> (118.3159, 14.957) centre (118.3184, 14.957) ccw
  arc A1010 (121.2719, 14.387) -> (121.2669, 14.387) centre (121.2694, 14.387) ccw
  arc A1011 (120.8089, 14.651) -> (120.8139, 14.651) centre (120.8114, 14.651) ccw
  arc A1012 (119.0299, 14.801) -> (119.0249, 14.801) centre (119.0274, 14.801) ccw
  arc A1013 (121.9099, 13.555) -> (121.9049, 13.555) centre (121.9074, 13.555) ccw
  arc A1014 (117.3799, 16.043) -> (117.3749, 16.043) centre (117.3774, 16.043) ccw
  arc A1015 (117.3799, 16.043) -> (117.3749, 16.043) centre (117.3774, 16.043) ccw
  arc A1016 (121.4659, 14.212) -> (121.4709, 14.212) centre (121.4684, 14.212) ccw
  arc A1017 (121.7929, 13.793) -> (121.7879, 13.793) centre (121.7904, 13.793) ccw
  arc A1018 (121.4659, 14.212) -> (121.4709, 14.212) centre (121.4684, 14.212) ccw
  arc A1019 (121.0509, 14.534) -> (121.0459, 14.534) centre (121.0484, 14.534) ccw
  arc A1020 (118.5519, 14.871) -> (118.5469, 14.871) centre (118.5494, 14.871) ccw
  arc A1021 (117.9009, 15.223) -> (117.9059, 15.223) centre (117.9034, 15.223) ccw
  arc A1022 (118.5519, 14.871) -> (118.5469, 14.871) centre (118.5494, 14.871) ccw
  arc A1023 (117.3269, 16.284) -> (117.3219, 16.284) centre (117.3244, 16.284) ccw
  arc A1024 (117.3049, 16.53) -> (117.3099, 16.53) centre (117.3074, 16.53) ccw
  arc A1025 (117.3269, 16.284) -> (117.3219, 16.284) centre (117.3244, 16.284) ccw
  line L267 (117.9034, 15.223) -> (118.1014, 15.075)
  arc A1026 (118.3159, 14.957) -> (118.3209, 14.957) centre (118.3184, 14.957) ccw
  arc A1027 (117.9059, 15.223) -> (117.9009, 15.223) centre (117.9034, 15.223) ccw
  arc A1028 (117.3799, 17.017) -> (117.3749, 17.017) centre (117.3774, 17.017) ccw
  line L268 (117.4634, 15.812) -> (117.5814, 15.595)
  arc A1029 (117.7269, 15.397) -> (117.7319, 15.397) centre (117.7294, 15.397) ccw
  arc A1030 (117.7319, 15.397) -> (117.7269, 15.397) centre (117.7294, 15.397) ccw
  arc A1031 (118.3209, 14.957) -> (118.3159, 14.957) centre (118.3184, 14.957) ccw
  arc A1032 (117.3219, 16.776) -> (117.3269, 16.776) centre (117.3244, 16.776) ccw
  arc A1033 (118.0989, 15.075) -> (118.1039, 15.075) centre (118.1014, 15.075) ccw
  arc A1034 (117.3219, 16.284) -> (117.3269, 16.284) centre (117.3244, 16.284) ccw
  arc A1035 (117.3269, 16.776) -> (117.3219, 16.776) centre (117.3244, 16.776) ccw
  arc A1036 (117.3749, 17.017) -> (117.3799, 17.017) centre (117.3774, 17.017) ccw
  arc A1037 (117.9059, 15.223) -> (117.9009, 15.223) centre (117.9034, 15.223) ccw
  arc A1038 (117.4659, 15.812) -> (117.4609, 15.812) centre (117.4634, 15.812) ccw
  line L269 (117.3074, 16.53) -> (117.3244, 16.776)
  arc A1039 (117.9009, 15.223) -> (117.9059, 15.223) centre (117.9034, 15.223) ccw
  arc A1040 (117.5839, 15.595) -> (117.5789, 15.595) centre (117.5814, 15.595) ccw
  line L270 (118.3184, 14.957) -> (118.5494, 14.871)
  arc A1041 (118.5469, 14.871) -> (118.5519, 14.871) centre (118.5494, 14.871) ccw
  arc A1042 (118.7929, 14.818) -> (118.7879, 14.818) centre (118.7904, 14.818) ccw
  arc A1043 (118.1039, 15.075) -> (118.0989, 15.075) centre (118.1014, 15.075) ccw
  arc A1044 (118.3159, 14.957) -> (118.3209, 14.957) centre (118.3184, 14.957) ccw
  arc A1045 (118.0989, 15.075) -> (118.1039, 15.075) centre (118.1014, 15.075) ccw
  arc A1046 (117.7269, 15.397) -> (117.7319, 15.397) centre (117.7294, 15.397) ccw
  arc A1047 (117.3269, 16.776) -> (117.3219, 16.776) centre (117.3244, 16.776) ccw
  arc A1048 (117.3749, 16.043) -> (117.3799, 16.043) centre (117.3774, 16.043) ccw
  arc A1049 (117.4609, 15.812) -> (117.4659, 15.812) centre (117.4634, 15.812) ccw
  line L271 (117.3074, 16.53) -> (117.3244, 16.284)
  arc A1050 (117.3219, 16.284) -> (117.3269, 16.284) centre (117.3244, 16.284) ccw
  arc A1051 (117.3049, 16.53) -> (117.3099, 16.53) centre (117.3074, 16.53) ccw
  line L272 (118.1014, 15.075) -> (118.3184, 14.957)
  arc A1052 (117.4609, 17.248) -> (117.4659, 17.248) centre (117.4634, 17.248) ccw
  line L273 (117.3774, 16.043) -> (117.4634, 15.812)
  arc A1053 (117.3099, 16.53) -> (117.3049, 16.53) centre (117.3074, 16.53) ccw
  arc A1054 (117.5839, 15.595) -> (117.5789, 15.595) centre (117.5814, 15.595) ccw
  line L274 (117.3244, 16.776) -> (117.3774, 17.017)
  arc A1055 (117.3219, 16.776) -> (117.3269, 16.776) centre (117.3244, 16.776) ccw
  arc A1056 (117.5789, 15.595) -> (117.5839, 15.595) centre (117.5814, 15.595) ccw
  arc A1057 (117.3749, 17.017) -> (117.3799, 17.017) centre (117.3774, 17.017) ccw
  line L275 (117.5814, 15.595) -> (117.7294, 15.397)
  line L276 (118.5494, 14.871) -> (118.7904, 14.818)
  arc A1058 (118.1039, 15.075) -> (118.0989, 15.075) centre (118.1014, 15.075) ccw
  arc A1059 (117.3799, 17.017) -> (117.3749, 17.017) centre (117.3774, 17.017) ccw
  line L277 (117.7294, 15.397) -> (117.9034, 15.223)
  arc A1060 (117.4659, 15.812) -> (117.4609, 15.812) centre (117.4634, 15.812) ccw
  arc A1061 (117.7319, 15.397) -> (117.7269, 15.397) centre (117.7294, 15.397) ccw
  arc A1062 (117.3099, 16.53) -> (117.3049, 16.53) centre (117.3074, 16.53) ccw
  arc A1063 (117.5789, 15.595) -> (117.5839, 15.595) centre (117.5814, 15.595) ccw
  arc A1064 (119.0389, 18.255) -> (119.0339, 18.255) centre (119.0364, 18.255) ccw
  arc A1065 (120.8139, 18.409) -> (120.8089, 18.409) centre (120.8114, 18.409) ccw
  line L278 (118.1014, 17.985) -> (118.3184, 18.103)
  arc A1066 (118.1039, 17.985) -> (118.0989, 17.985) centre (118.1014, 17.985) ccw
  arc A1067 (118.5519, 18.189) -> (118.5469, 18.189) centre (118.5494, 18.189) ccw
  arc A1068 (120.5629, 18.324) -> (120.5579, 18.324) centre (120.5604, 18.324) ccw
  line L279 (120.3004, 18.272) -> (120.5604, 18.324)
  line L280 (117.3774, 17.017) -> (117.4634, 17.248)
  arc A1069 (120.0339, 18.255) -> (120.0389, 18.255) centre (120.0364, 18.255) ccw
  arc A1070 (120.5579, 18.324) -> (120.5629, 18.324) centre (120.5604, 18.324) ccw
  arc A1071 (119.0299, 18.259) -> (119.0249, 18.259) centre (119.0274, 18.259) ccw
  arc A1072 (117.7269, 17.663) -> (117.7319, 17.663) centre (117.7294, 17.663) ccw
  arc A1073 (118.7929, 18.242) -> (118.7879, 18.242) centre (118.7904, 18.242) ccw
  line L281 (119.0364, 18.255) -> (120.0364, 18.255)
  arc A1074 (117.9059, 17.837) -> (117.9009, 17.837) centre (117.9034, 17.837) ccw
  arc A1075 (120.3029, 18.272) -> (120.2979, 18.272) centre (120.3004, 18.272) ccw
  arc A1076 (120.5579, 18.324) -> (120.5629, 18.324) centre (120.5604, 18.324) ccw
  arc A1077 (120.0389, 18.255) -> (120.0339, 18.255) centre (120.0364, 18.255) ccw